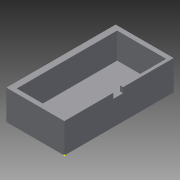
# Autodesk Inventor part: caixav2
Saved by Autodesk Inventor 2013 SP2 (Build 170200200, 200)
## iProperties
Created: 2017-01-18
Part Number: caixav2
Material: Generic
Document SubType Name: Modeling
Designer: 12el18
Density: 1 g/cm^3
Author: 12el18
Autodesk Inventor part; units mm, degrees
ref_plane "YZ Plane" through (0, 0, 0) normal (1, 0, 0) x (0, 1, 0)
ref_plane "XZ Plane" through (0, 0, 0) normal (0, 1, 0) x (-1, 0, 0)
ref_plane "XY Plane" through (0, 0, 0) normal (0, 0, 1) x (1, 0, 0)
sketch "Sketch1" plane through (0, 0, 0) normal (0, 1, 0) x (-1, 0, 0)
  point P0 (0, 0)
sketch "Sketch2" plane through (0, 0, 0) normal (0, 1, 0) x (-1, 0, 0)
  line L0 (0, 0) -> (0, -147)
  line L1 (0, -147) -> (78, -147)
  line L2 (78, -147) -> (78, 0)
  line L3 (78, 0) -> (0, 0)
  dimension "d0" = 147
  dimension "d1" = 78
  constraints: 8 end point, 2 parallel, 1 perpendicular, 1 vertical
  measures "d0" distance of L0.start L0.end
  measures "d1" distance of L0.end L1.end
extrude "Extrusion1" add sketch "Sketch2" along normal blind 5
sketch "Sketch3" plane through (0, 5, 0) normal (0, 1, 0) x (1, 0, 0)
  line L0 (0, 0) -> (0, 147) projected
  line L1 (-78, 0) -> (0, 0) projected
  line L2 (0, 0) -> (-4, 0)
  line L3 (-4, 0) -> (-4, 66)
  line L4 (-4, 66) -> (0, 66)
  dimension "d4" = 4
  dimension "d5" = 66
  constraints: 6 end point, 2 point on line, 1 parallel, 1 perpendicular
  measures "d4" distance of L0.start L2.end
  measures "d5" distance of L2.end L3.end
extrude "Extrusion2" add sketch "Sketch3" along normal blind 35
sketch "Sketch4" plane through (0, 5, 0) normal (0, 1, 0) x (1, 0, 0)
  line L0 (-4, 66) -> (0, 66) projected
  line L1 (0, 66) -> (0, 147) projected
  line L2 (0, 66) -> (0, 79)
  line L3 (0, 79) -> (-4, 79)
  line L4 (-4, 79) -> (-4, 66)
  point P0 (0, 0)
  dimension "d8" = 13
  constraints: 6 end point, 1 parallel, 1 perpendicular, 1 point on line
  measures "d8" distance of L0.end L2.end
extrude "Extrusion3" add sketch "Sketch4" along normal blind 28
sketch "Sketch5" plane through (0, 5, 0) normal (0, 1, 0) x (1, 0, 0)
  line L0 (-4, 79) -> (0, 79) projected
  line L1 (0, 79) -> (0, 147) projected
  line L2 (0, 147) -> (-78, 147) projected
  line L3 (-4, 79) -> (-4, 147)
  line L4 (0, 147) -> (0, 79)
  point P0 (0, 0)
  constraints: 4 end point, 1 collinear, 1 perpendicular, 1 point on line
extrude "Extrusion4" add sketch "Sketch5" along normal blind 35
sketch "Sketch6" plane through (0, 5, 0) normal (0, 1, 0) x (1, 0, 0)
  line L0 (-4, 0) -> (-4, 147) projected
  line L1 (-4, 147) -> (-78, 147) projected
  line L2 (-78, 147) -> (-78, 0) projected
  line L3 (-4, 147) -> (-4, 141)
  line L4 (-4, 141) -> (-78, 141)
  line L5 (-78, 147) -> (-4, 147)
  point P0 (0, 0)
  dimension "d13" = 6
  constraints: 6 end point, 2 point on line, 1 collinear, 1 perpendicular
  measures "d13" distance of L0.end L3.end
extrude "Extrusion5" add sketch "Sketch6" along normal blind 35
sketch "Sketch7" plane through (0, 5, 0) normal (0, 1, 0) x (1, 0, 0)
  line L0 (-4, 141) -> (-78, 141) projected
  line L1 (-78, 141) -> (-78, 0) projected
  line L2 (-78, 0) -> (-4, 0) projected
  line L3 (-78, 141) -> (-78, 0)
  line L4 (-78, 0) -> (-70, 0)
  line L5 (-70, 0) -> (-70, 141)
  point P0 (0, 0)
  dimension "d16" = 8
  constraints: 6 end point, 2 point on line, 1 collinear, 1 perpendicular
  measures "d16" distance of L1.end L4.end
extrude "Extrusion6" add sketch "Sketch7" along normal blind 35
sketch "Sketch8" plane through (0, 5, 0) normal (0, 1, 0) x (1, 0, 0)
  line L0 (-70, 141) -> (-70, 0) projected
  line L1 (-70, 0) -> (-4, 0) projected
  line L2 (-4, 0) -> (-4, 141) projected
  line L3 (-4, 141) -> (-70, 141) projected
  line L4 (-4, 0) -> (-70, 0)
  line L5 (-4, 0) -> (-4, 6)
  line L6 (-4, 6) -> (-70, 6)
  point P0 (0, 0)
  dimension "d19" = 6
  constraints: 6 end point, 2 point on line, 1 parallel, 1 perpendicular
  measures "d19" distance of L1.end L5.end
extrude "Extrusion7" add sketch "Sketch8" along normal blind 35 contours L6 L2 L1 L0
body "Solid1"
